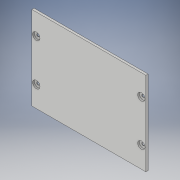
# Autodesk Inventor part: Ra-Manager_Painel-Placas_Tras_Cego
Saved by Autodesk Inventor 2019.4 (Build 234330000, 330)
## iProperties
Created: 2020-03-24
Part Number: Ra-Manager_Painel-Placas_Tras_Cego
Material: Genérico
Document SubType Name: Modeling
Designer: caiom
Density: 1 g/cm^3
Appearance: Padrão
Author: caiom
Autodesk Inventor part; units mm, degrees
ref_plane "YZ Plane" through (0, 0, 0) normal (1, 0, 0) x (0, 1, 0)
ref_plane "XZ Plane" through (0, 0, 0) normal (0, 1, 0) x (-1, 0, 0)
ref_plane "XY Plane" through (0, 0, 0) normal (0, 0, 1) x (1, 0, 0)
sketch "Esboço1" plane through (0, 0, 0) normal (0, 0, 1) x (1, 0, 0)
  line L0 (-50.5, -37) -> (50.5, -37)
  line L1 (50.5, -37) -> (50.5, 37)
  line L2 (50.5, 37) -> (-50.5, 37)
  line L3 (-50.5, 37) -> (-50.5, -37)
  point P0 (0, 0)
  dimension "d2" = 101
  dimension "d3" = 74
  dimension "d4" = 101
  dimension "d5" = 50.5
  dimension "d6" = 37
  constraints: 8 end point, 1 parallel, 1 perpendicular, 1 vertical
  measures "d2" distance of L0.start L0.end
  measures "d3" distance of L0.end L1.end
  measures "d4" distance of L1.end L2.end
  measures "d5" distance from line of point (0, 0) L1
  measures "d6" distance from line of point (0, 0) L2
extrude "Extrusão1" add sketch "Esboço1" against normal blind 2
sketch "Esboço2" plane through (0, 0, 0) normal (0, 0, 1) x (1, 0, 0)
  line L0 (-50.5, -37) -> (-50.5, 37) projected
  line L1 (-50.5, 37) -> (50.5, 37) projected
  line L2 (-46.5, 37) -> (-46.5, -37) construction
  line L3 (50.5, -37) -> (-50.5, -37) projected
  line L4 (46.5, 37) -> (46.5, -37) construction
  line L5 (-50.5, 18.5) -> (50.5, 18.5) construction
  line L6 (-50.5, -18.5) -> (50.5, -18.5) construction
  line L7 (50.5, 37) -> (50.5, -37) projected
  point P0 (0, 0)
  point P1 (-46.5, 18.5)
  point P2 (-46.5, -18.5)
  point P3 (46.5, -18.5)
  point P4 (46.5, 18.5)
  dimension "d13" = 4
  dimension "d14" = 97
  dimension "d15" = 18.5
  dimension "d16" = 55.5
  dimension "d17" = 0
  constraints: 15 point on line, 8 end point, 2 horizontal, 1 parallel, 1 perpendicular
  measures "d13" distance between parallel lines of L7 L4
  measures "d14" distance between parallel lines of L7 L2
  measures "d15" distance between parallel lines of L1 L5
  measures "d16" distance between parallel lines of L1 L6
  measures "d17" distance from line of L5.end L7
hole "Furo1" at (-46.5, 18.5, 0) at (-46.5, -18.5, 0) at (46.5, -18.5, 0) at (46.5, 18.5, 0) direction (0, 0, -1) diameter 2.459 end through all counterbore diameter 6.5 counterbore depth 1.5 thread size "M3x0.5" class "6H" standard "ANSI Metric M Profile"
